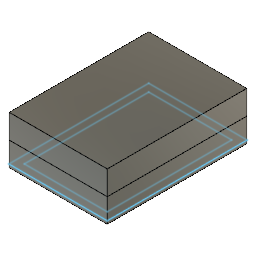
pin_box2 (Autodesk Fusion 360 design; units mm, degrees)
Autodesk Fusion 360 part; units mm, degrees
sketch "Sketch1" plane through (0, 0, 0) normal (0, 0, 1) x (1, 0, 0)
  line L0 (-20, 30) -> (27.4, 30)
  line L1 (27.4, 30) -> (27.4, -37.4)
  line L2 (27.4, -37.4) -> (-20, -37.4)
  line L3 (-20, -37.4) -> (-20, 30)
  line L4 (-16.3, 26.3) -> (23.7, 26.3)
  line L5 (23.7, 26.3) -> (23.7, -33.7)
  line L6 (23.7, -33.7) -> (-16.3, -33.7)
  line L7 (-16.3, -33.7) -> (-16.3, 26.3)
  dimension "d1" = 47.4
  dimension "d2" = 67.4
  dimension "d3" = 40
  dimension "d4" = 60
  dimension "d5" = 3.7
  dimension "d6" = 3.7
  constraint horizontal L0
  constraint vertical L1
  constraint horizontal L2
  constraint vertical L3
  constraint horizontal L4
  constraint vertical L5
  constraint horizontal L6
  constraint vertical L7
  measures "d1" distance of L0.start L0.end
  measures "d2" distance of L0.start L2.end
  measures "d3" distance of L4.start L4.end
  measures "d4" distance of L4.start L6.end
  measures "d5" distance of L0 L4
  measures "d6" distance of L3 L7
extrude "Extrude1" add sketch "Sketch1" against normal blind 1.6 contours L0 L1 L2 L3 | L4 L5 L6 L7 makes body 1
copy_body "Body->Comp1" bodies 1 removing the originals makes body 2 in component "Component"
extrude "Extrude1'" add sketch "Sketch1" along normal blind 10 bodies 2 in component "Component"
sketch "Sketch1 (2)" plane through (0, 0, 10) normal (0, 0, 1) x (-1, 0, 0) in component "Component"
  line L0 (-23.7, 33.7) -> (16.3, 33.7)
  line L1 (16.3, 33.7) -> (16.3, -26.3)
  line L2 (16.3, -26.3) -> (-23.7, -26.3)
  line L3 (-23.7, -26.3) -> (-23.7, 33.7)
  line L4 (20, 37.4) -> (-27.4, 37.4)
  line L5 (-27.4, 37.4) -> (-27.4, -30)
  line L6 (-27.4, -30) -> (20, -30)
  line L7 (20, -30) -> (20, 37.4)
  line L8 (16.3, -26.3) -> (-23.7, -26.3)
  line L9 (-23.7, -26.3) -> (-23.7, 33.7)
  line L10 (-23.7, 33.7) -> (16.3, 33.7)
  line L11 (16.3, 33.7) -> (16.3, -26.3)
  line L12 (17.9, 0.1212) -> (18.4, 0.1212)
  line L13 (18.4, 0.1212) -> (18.4, 4.1212)
  line L14 (18.4, 4.1212) -> (17.9, 4.1212)
  line L15 (17.9, 35.3) -> (17.9, 4.1212)
  line L16 (17.9, 0.1212) -> (17.9, -27.9)
  line L17 (-25.3, 0.0803) -> (-25.8, 0.0803)
  line L18 (-25.8, 0.0803) -> (-25.8, 4.0803)
  line L19 (-25.8, 4.0803) -> (-25.3, 4.0803)
  line L20 (-25.3, -27.9) -> (-25.3, 0.0803)
  line L21 (-25.3, 4.0803) -> (-25.3, 35.3)
  line L22 (-5.1137, -27.9) -> (-5.1137, -28.4)
  line L23 (-5.1137, -28.4) -> (-2.1137, -28.4)
  line L24 (-2.1137, -28.4) -> (-2.1137, -27.9)
  line L25 (17.9, -27.9) -> (-2.1137, -27.9)
  line L26 (-5.1137, -27.9) -> (-25.3, -27.9)
  line L27 (-5.243, 35.3) -> (-5.243, 35.8)
  line L28 (-5.243, 35.8) -> (-2.243, 35.8)
  line L29 (-2.243, 35.8) -> (-2.243, 35.3)
  line L30 (-25.3, 35.3) -> (-5.243, 35.3)
  line L31 (-2.243, 35.3) -> (17.9, 35.3)
  dimension "d11" = 43.2
  dimension "d12" = 63.2
  dimension "d13" = 1.6
  dimension "d14" = 1.6
  dimension "d15" = 0.5
  dimension "d16" = 4
  dimension "d17" = 0.5
  dimension "d18" = 4
  dimension "d19" = 3
  dimension "d20" = 0.5
  dimension "d21" = 3
  dimension "d22" = 0.5
  constraint horizontal L8
  constraint vertical L9
  constraint horizontal L10
  constraint vertical L11
  constraint coincident L0.start L3.end
  constraint coincident L1.end L2.start
  constraint horizontal L25
  constraint vertical L20
  constraint horizontal L30
  constraint vertical L15
  constraint horizontal L12
  constraint vertical L13
  constraint horizontal L14
  constraint coincident L12.start L15
  constraint collinear L15 L16
  constraint horizontal L17
  constraint vertical L18
  constraint horizontal L19
  constraint collinear L20 L21
  constraint vertical L22
  constraint horizontal L23
  constraint vertical L24
  constraint collinear L25 L26
  constraint vertical L27
  constraint horizontal L28
  constraint vertical L29
  constraint coincident L29.end L30
  constraint collinear L30 L31
  measures "d11" distance of L16.end L20.start
  measures "d12" distance of L16.end L15.start
  measures "d13" distance of L11 L15
  measures "d14" distance of L8 L25
  measures "d15" distance of L12.start L12.end
  measures "d16" distance of L12.start L14.end
  measures "d17" distance of L17.start L17.end
  measures "d18" distance of L17.start L19.end
  measures "d19" distance of L24.end L22.start
  measures "d20" distance of L24.end L23.end
  measures "d21" distance of L29.end L27.start
  measures "d22" distance of L29.end L28.end
extrude "Extrude2" add sketch "Sketch1 (2)" along normal blind 10 contours L12 L13 L14 L15 L16 L17 L18 L19 L20 L21 L22 L23 L24 L25 L26 L27 L28 L29 L30 L31 bodies 2 in component "Component"
sketch "Sketch2" plane through (0, 0, 10) normal (0, 0, 1) x (-1, 0, 0) in component "Component"
  line L0 (-5.1137, -27.9) -> (-25.3, -27.9)
  line L1 (-25.3, -27.9) -> (-25.3, 0.0803)
  line L2 (-25.3, 0.0803) -> (-25.8, 0.0803)
  line L3 (-25.8, 0.0803) -> (-25.8, 4.0803)
  line L4 (-25.8, 4.0803) -> (-25.3, 4.0803)
  line L5 (-25.3, 4.0803) -> (-25.3, 35.3)
  line L6 (-25.3, 35.3) -> (-5.243, 35.3)
  line L7 (-5.243, 35.3) -> (-5.243, 35.8)
  line L8 (-5.243, 35.8) -> (-2.243, 35.8)
  line L9 (-2.243, 35.8) -> (-2.243, 35.3)
  line L10 (-2.243, 35.3) -> (17.9, 35.3)
  line L11 (17.9, 35.3) -> (17.9, 4.1212)
  line L12 (17.9, 4.1212) -> (18.4, 4.1212)
  line L13 (18.4, 4.1212) -> (18.4, 0.1212)
  line L14 (18.4, 0.1212) -> (17.9, 0.1212)
  line L15 (17.9, 0.1212) -> (17.9, -27.9)
  line L16 (17.9, -27.9) -> (-2.1137, -27.9)
  line L17 (-2.1137, -27.9) -> (-2.1137, -28.4)
  line L18 (-2.1137, -28.4) -> (-5.1137, -28.4)
  line L19 (-5.1137, -28.4) -> (-5.1137, -27.9)
  line L20 (20, 37.4) -> (-27.4, 37.4)
  line L21 (-27.4, 37.4) -> (-27.4, -30)
  line L22 (-27.4, -30) -> (20, -30)
  line L23 (20, -30) -> (20, 37.4)
  line L24 (20, -30) -> (-27.4, -30)
  line L25 (-27.4, -30) -> (-27.4, 37.4)
  line L26 (-27.4, 37.4) -> (20, 37.4)
  line L27 (20, 37.4) -> (20, -30)
  line L28 (18.4, -28.4) -> (-25.8, -28.4)
  line L29 (-25.8, -28.4) -> (-25.8, 35.8)
  line L30 (-25.8, 35.8) -> (18.4, 35.8)
  line L31 (18.4, 35.8) -> (18.4, -28.4)
  dimension "d25" = 44.2
  dimension "d26" = 64.2
  dimension "d27" = 1.6
  dimension "d28" = 1.6
  constraint horizontal L24
  constraint vertical L25
  constraint horizontal L26
  constraint vertical L27
  constraint coincident L20.end L21.start
  constraint coincident L22.end L23.start
  constraint horizontal L28
  constraint vertical L29
  constraint horizontal L30
  constraint vertical L31
  measures "d25" distance of L28.start L28.end
  measures "d26" distance of L28.start L30.end
  measures "d27" distance of L27 L31
  measures "d28" distance of L24 L28
extrude "Extrude1''" add sketch "Sketch2" along normal blind 10 separate body makes body 3 in component "Component'"
sketch "Sketch1 (3)" plane through (0, 0, 20) normal (0, 0, 1) x (-1, 0, 0) in component "Component'"
  line L0 (-25.8, 35.8) -> (18.4, 35.8)
  line L1 (18.4, 35.8) -> (18.4, -28.4)
  line L2 (18.4, -28.4) -> (-25.8, -28.4)
  line L3 (-25.8, -28.4) -> (-25.8, 35.8)
  line L4 (20, 37.4) -> (-27.4, 37.4)
  line L5 (-27.4, 37.4) -> (-27.4, -30)
  line L6 (-27.4, -30) -> (20, -30)
  line L7 (20, -30) -> (20, 37.4)
  line L8 (20, -30) -> (-27.4, -30)
  line L9 (-27.4, -30) -> (-27.4, 37.4)
  line L10 (-27.4, 37.4) -> (20, 37.4)
  line L11 (20, 37.4) -> (20, -30)
  constraint horizontal L8
  constraint vertical L9
  constraint horizontal L10
  constraint vertical L11
  constraint coincident L4.end L5.start
  constraint coincident L6.end L7.start
extrude "Extrude2'" add sketch "Sketch1 (3)" along normal blind 1.6 contours L0 L1 L2 L3 | L4 L5 L6 L7 L8 L9 L10 L11 bodies 3 in component "Component'"
component "Component" placed x (1, 0, 0) y (0, 1, 0) z (0, 0, 1) at (0, 0, 0)
component "Component'" placed x (1, 0, 0) y (0, 1, 0) z (0, 0, 1) at (0, 0, 0) in component "Component"
